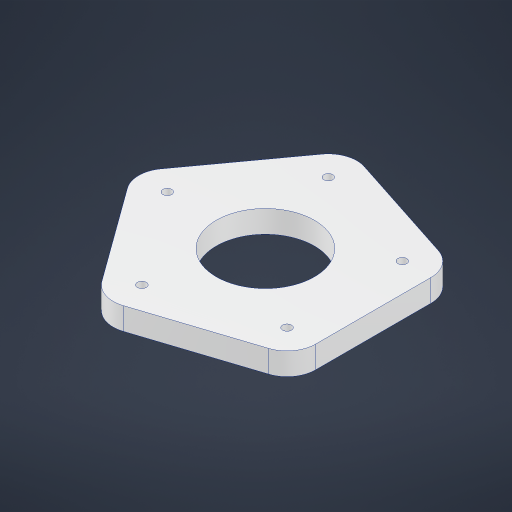
# Autodesk Inventor part: gearSpacer
Saved by Autodesk Inventor 2023.2 (Build 272271030, 271C)
## iProperties
Created: 2023-01-27
Part Number: gearSpacer
Material: Aluminum 6061
Document SubType Name: Modeling
Designer: kumpu
Density: 2.7 g/cm^3
Appearance: Aluminum - Flat
Author: kumpu
Autodesk Inventor part; units mm, degrees
ref_plane "YZ Plane" through (0, 0, 0) normal (1, 0, 0) x (0, 1, 0)
ref_plane "XZ Plane" through (0, 0, 0) normal (0, 1, 0) x (-1, 0, 0)
ref_plane "XY Plane" through (0, 0, 0) normal (0, 0, 1) x (1, 0, 0)
sketch "Sketch1" plane through (0, 0, 0) normal (0, 1, 0) x (-1, 0, 0)
  circle A0 centre (0, 0) radius 19.304
  line L0 (0, 0) -> (27.94, 0) construction
  circle A1 centre (27.94, 0) radius 3.3782
  circle A2 centre (8.6339, 26.5725) radius 3.3782
  circle A3 centre (-22.6039, 16.4227) radius 3.3782
  circle A4 centre (-22.6039, -16.4227) radius 3.3782
  circle A5 centre (8.6339, -26.5725) radius 3.3782
  line L1 (34.526, 4.785) -> (15.2199, 31.3575)
  arc A6 (15.2199, 31.3575) -> (6.1183, 34.3148) centre (8.6339, 26.5725) ccw
  line L2 (6.1183, 34.3148) -> (-25.1195, 24.165)
  arc A7 (-25.1195, 24.165) -> (-30.7446, 16.4227) centre (-22.6039, 16.4227) ccw
  line L3 (-30.7446, 16.4227) -> (-30.7446, -16.4227)
  arc A8 (-30.7446, -16.4227) -> (-25.1195, -24.165) centre (-22.6039, -16.4227) ccw
  line L4 (-25.1195, -24.165) -> (6.1183, -34.3148)
  arc A9 (6.1183, -34.3148) -> (15.2199, -31.3575) centre (8.6339, -26.5725) ccw
  line L5 (15.2199, -31.3575) -> (34.526, -4.785)
  arc A10 (34.526, -4.785) -> (34.526, 4.785) centre (27.94, 0) ccw
  dimension "d0" = 38.608
  dimension "d1" = 27.94
  dimension "d2" = 6.7564
  dimension "d5" = 360
  dimension "d7" = 4.7625
  constraints: 12 end point, 11 centre point, 10 point on circle, 10 tangent, 5 concentric, 4 equal radius, 2 coincident, 1 horizontal, 11 other
  measures "d0" diameter of A0
  measures "d1" distance of L0.start L0.end
  measures "d2" diameter of A1
  measures "d7" radial gap between concentric circles of A1 A10
extrude "Extrusion1" add sketch "Sketch1" along normal blind 6.35
sketch "Sketch2" plane through (0, 6.35, 0) normal (0, 1, 0) x (1, 0, 0)
  arc A0 (-15.2199, -31.3575) -> (-6.1183, -34.3148) centre (-8.6339, -26.5725) ccw projected
  line L0 (-6.1183, -34.3148) -> (25.1195, -24.165) projected
  arc A1 (25.1195, -24.165) -> (30.7446, -16.4227) centre (22.6039, -16.4227) ccw projected
  line L1 (30.7446, -16.4227) -> (30.7446, 16.4227) projected
  arc A2 (30.7446, 16.4227) -> (25.1195, 24.165) centre (22.6039, 16.4227) ccw projected
  line L2 (25.1195, 24.165) -> (-6.1183, 34.3148) projected
  arc A3 (-6.1183, 34.3148) -> (-15.2199, 31.3575) centre (-8.6339, 26.5725) ccw projected
  line L3 (-15.2199, 31.3575) -> (-34.526, 4.785) projected
  arc A4 (-34.526, 4.785) -> (-34.526, -4.785) centre (-27.94, 0) ccw projected
  line L4 (-34.526, -4.785) -> (-15.2199, -31.3575) projected
  circle A5 centre (-27.94, 0) radius 3.3782 projected
  circle A6 centre (-8.6339, 26.5725) radius 3.3782 projected
  circle A7 centre (22.6039, 16.4227) radius 3.3782 projected
  circle A8 centre (22.6039, -16.4227) radius 3.3782 projected
  circle A9 centre (-8.6339, -26.5725) radius 3.3782 projected
  circle A10 centre (0, 0) radius 19.304 projected
  circle A11 centre (0, 0) radius 13.97
  circle A12 centre (-27.94, 0) radius 1.27
  circle A13 centre (-8.6339, 26.5725) radius 1.27
  circle A14 centre (22.6039, 16.4227) radius 1.27
  circle A15 centre (22.6039, -16.4227) radius 1.27
  circle A16 centre (-8.6339, -26.5725) radius 1.27
  dimension "d10" = 27.94
  dimension "d11" = 2.54
  dimension "d12" = 2.54
  dimension "d13" = 2.54
  dimension "d14" = 2.54
  dimension "d15" = 2.54
  constraints: 6 centre point, 6 coincident
  measures "d10" diameter of A11
  measures "d11" diameter of A12
  measures "d12" diameter of A13
  measures "d13" diameter of A14
  measures "d14" diameter of A15
  measures "d15" diameter of A16
extrude "Extrusion2" add sketch "Sketch2" against normal up to surface (6.35 mm away) contours A5 | A6 | A7 | A8 | A9 | A10
body "Solid1"
